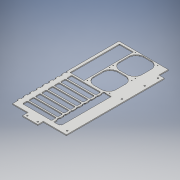
# Autodesk Inventor part: backpanel2
Saved by Autodesk Inventor 2018 (Build 220112000, 112)
## iProperties
Created: 2021-05-09
Part Number: backpanel2
Material: Generic
Document SubType Name: Modeling
Designer: gisen
Density: 1 g/cm^3
Appearance: Default
Author: gisen
Autodesk Inventor part; units mm, degrees
(part 1 of 2)
ref_plane "YZ Plane" through (0, 0, 0) normal (1, 0, 0) x (0, 1, 0)
ref_plane "XZ Plane" through (0, 0, 0) normal (0, 1, 0) x (-1, 0, 0)
ref_plane "XY Plane" through (0, 0, 0) normal (0, 0, 1) x (1, 0, 0)
sketch "Sketch2" plane through (0, 0, 0) normal (0, 0, 1) x (1, 0, 0)
  arc A0 (64.4142, -110.1237) -> (63.7071, -110.4166) centre (64.4142, -111.1237) ccw
  line L0 (63.7071, -110.4166) -> (59.2929, -114.8308)
  arc A1 (58.5858, -115.1237) -> (59.2929, -114.8308) centre (58.5858, -114.1237) ccw
  line L1 (58.5858, -115.1237) -> (43.2196, -115.1237)
  arc A2 (42.2196, -114.1237) -> (43.2196, -115.1237) centre (43.2196, -114.1237) ccw
  line L2 (42.2196, -114.1237) -> (42.2196, -104.6674)
  arc A3 (42.2196, -104.6674) -> (40.773, -102.7455) centre (40.2196, -104.6674) ccw
  arc A4 (39.7673, -102.1811) -> (40.773, -102.7455) centre (41.4696, -100.3262) ccw
  arc A5 (39.1196, -100.7076) -> (39.7673, -102.1811) centre (41.1196, -100.7076) ccw
  line L3 (39.1196, -100.7076) -> (39.1196, -95.7515)
  arc A6 (39.7673, -94.2779) -> (39.1196, -95.7515) centre (41.1196, -95.7515) ccw
  arc A7 (39.937, -94.1354) -> (39.7673, -94.2779) centre (41.4696, -96.1328) ccw
  arc A8 (39.937, -94.1354) -> (40.7196, -92.5486) centre (38.7196, -92.5486) ccw
  line L4 (40.7196, -92.5486) -> (40.7196, -83.4104)
  arc A9 (40.7196, -83.4104) -> (39.937, -81.8236) centre (38.7196, -83.4104) ccw
  arc A10 (39.7673, -81.6811) -> (39.937, -81.8236) centre (41.4696, -79.8262) ccw
  arc A11 (39.1196, -80.2076) -> (39.7673, -81.6811) centre (41.1196, -80.2076) ccw
  line L5 (39.1196, -80.2076) -> (39.1196, -75.2515)
  arc A12 (39.7673, -73.7779) -> (39.1196, -75.2515) centre (41.1196, -75.2515) ccw
  arc A13 (39.937, -73.6354) -> (39.7673, -73.7779) centre (41.4696, -75.6328) ccw
  arc A14 (39.937, -73.6354) -> (40.7196, -72.0486) centre (38.7196, -72.0486) ccw
  line L6 (40.7196, -72.0486) -> (40.7196, -62.9104)
  arc A15 (40.7196, -62.9104) -> (39.937, -61.3236) centre (38.7196, -62.9104) ccw
  arc A16 (39.7673, -61.1811) -> (39.937, -61.3236) centre (41.4696, -59.3262) ccw
  arc A17 (39.1196, -59.7076) -> (39.7673, -61.1811) centre (41.1196, -59.7076) ccw
  line L7 (39.1196, -59.7076) -> (39.1196, -54.7515)
  arc A18 (39.7673, -53.2779) -> (39.1196, -54.7515) centre (41.1196, -54.7515) ccw
  arc A19 (39.937, -53.1354) -> (39.7673, -53.2779) centre (41.4696, -55.1328) ccw
  arc A20 (39.937, -53.1354) -> (40.7196, -51.5486) centre (38.7196, -51.5486) ccw
  line L8 (40.7196, -51.5486) -> (40.7196, -42.4104)
  arc A21 (40.7196, -42.4104) -> (39.937, -40.8236) centre (38.7196, -42.4104) ccw
  arc A22 (39.7673, -40.6811) -> (39.937, -40.8236) centre (41.4696, -38.8262) ccw
  arc A23 (39.1196, -39.2076) -> (39.7673, -40.6811) centre (41.1196, -39.2076) ccw
  line L9 (39.1196, -39.2076) -> (39.1196, -34.2515)
  arc A24 (39.7673, -32.7779) -> (39.1196, -34.2515) centre (41.1196, -34.2515) ccw
  arc A25 (39.937, -32.6354) -> (39.7673, -32.7779) centre (41.4696, -34.6328) ccw
  arc A26 (39.937, -32.6354) -> (40.7196, -31.0486) centre (38.7196, -31.0486) ccw
  line L10 (40.7196, -31.0486) -> (40.7196, -21.9104)
  arc A27 (40.7196, -21.9104) -> (39.937, -20.3236) centre (38.7196, -21.9104) ccw
  arc A28 (39.7673, -20.1811) -> (39.937, -20.3236) centre (41.4696, -18.3262) ccw
  arc A29 (39.1196, -18.7076) -> (39.7673, -20.1811) centre (41.1196, -18.7076) ccw
  line L11 (39.1196, -18.7076) -> (39.1196, -13.7515)
  arc A30 (39.7673, -12.2779) -> (39.1196, -13.7515) centre (41.1196, -13.7515) ccw
  arc A31 (39.937, -12.1354) -> (39.7673, -12.2779) centre (41.4696, -14.1328) ccw
  arc A32 (39.937, -12.1354) -> (40.7196, -10.5486) centre (38.7196, -10.5486) ccw
  line L12 (40.7196, -10.5486) -> (40.7196, -1.4104)
  arc A33 (40.7196, -1.4104) -> (39.937, 0.1764) centre (38.7196, -1.4104) ccw
  arc A34 (39.7673, 0.3189) -> (39.937, 0.1764) centre (41.4696, 2.1738) ccw
  arc A35 (39.1196, 1.7924) -> (39.7673, 0.3189) centre (41.1196, 1.7924) ccw
  line L13 (39.1196, 1.7924) -> (39.1196, 6.7485)
  arc A36 (39.7673, 8.2221) -> (39.1196, 6.7485) centre (41.1196, 6.7485) ccw
  arc A37 (39.937, 8.3646) -> (39.7673, 8.2221) centre (41.4696, 6.3672) ccw
  arc A38 (39.937, 8.3646) -> (40.7196, 9.9514) centre (38.7196, 9.9514) ccw
  line L14 (40.7196, 9.9514) -> (40.7196, 19.0896)
  arc A39 (40.7196, 19.0896) -> (39.937, 20.6764) centre (38.7196, 19.0896) ccw
  arc A40 (39.7673, 20.8189) -> (39.937, 20.6764) centre (41.4696, 22.6738) ccw
  arc A41 (39.1196, 22.2924) -> (39.7673, 20.8189) centre (41.1196, 22.2924) ccw
  line L15 (39.1196, 22.2924) -> (39.1196, 27.2485)
  arc A42 (39.7673, 28.7221) -> (39.1196, 27.2485) centre (41.1196, 27.2485) ccw
  arc A43 (39.937, 28.8646) -> (39.7673, 28.7221) centre (41.4696, 26.8672) ccw
  arc A44 (39.937, 28.8646) -> (40.7196, 30.4514) centre (38.7196, 30.4514) ccw
  line L16 (40.7196, 30.4514) -> (40.7196, 39.5896)
  arc A45 (40.7196, 39.5896) -> (39.937, 41.1764) centre (38.7196, 39.5896) ccw
  arc A46 (39.7673, 41.3189) -> (39.937, 41.1764) centre (41.4696, 43.1738) ccw
  arc A47 (39.1196, 42.7924) -> (39.7673, 41.3189) centre (41.1196, 42.7924) ccw
  line L17 (39.1196, 42.7924) -> (39.1196, 47.7485)
  arc A48 (39.7673, 49.2221) -> (39.1196, 47.7485) centre (41.1196, 47.7485) ccw
  arc A49 (43.3362, 49.0566) -> (39.7673, 49.2221) centre (41.4696, 47.3672) ccw
  arc A50 (43.3362, 49.0566) -> (44.819, 48.3987) centre (44.819, 50.3987) ccw
  line L18 (44.819, 48.3987) -> (75, 48.3987)
  line L19 (75, 48.3987) -> (75, 184.5)
  line L20 (75, 184.5) -> (57.5, 184.5)
  line L21 (57.5, 184.5) -> (57.5, 215)
  line L22 (57.5, 215) -> (55, 215)
  line L23 (55, 215) -> (55, 220)
  line L24 (55, 220) -> (24.5, 220)
  line L25 (24.5, 220) -> (24.5, 232.5)
  line L26 (24.5, 232.5) -> (-24.5, 232.5)
  line L27 (-24.5, 232.5) -> (-24.5, 220)
  line L28 (-24.5, 220) -> (-55, 220)
  line L29 (-55, 220) -> (-55, 215)
  line L30 (-55, 215) -> (-78, 215)
  line L31 (-78, 215) -> (-78, 46.0635)
  line L32 (-78, 46.0635) -> (-75, 46.0635)
  line L33 (-75, 46.0635) -> (-75, 40.8932)
  line L34 (-75, 40.8932) -> (-78, 40.8932)
  line L35 (-78, 40.8932) -> (-78, 30.6062)
  line L36 (-78, 30.6062) -> (-75, 30.6062)
  line L37 (-75, 30.6062) -> (-75, 20.5478)
  line L38 (-75, 20.5478) -> (-78, 20.5478)
  line L39 (-78, 20.5478) -> (-78, 10.2608)
  line L40 (-78, 10.2608) -> (-75, 10.2608)
  line L41 (-75, 10.2608) -> (-75, -0.1068)
  line L42 (-75, -0.1068) -> (-78, -0.1068)
  line L43 (-78, -0.1068) -> (-78, -10.3938)
  line L44 (-78, -10.3938) -> (-75, -10.3938)
  line L45 (-75, -10.3938) -> (-75, -20.4522)
  line L46 (-75, -20.4522) -> (-78, -20.4522)
  line L47 (-78, -20.4522) -> (-78, -30.7392)
  line L48 (-78, -30.7392) -> (-75, -30.7392)
  line L49 (-75, -30.7392) -> (-75, -41.1068)
  line L50 (-75, -41.1068) -> (-78, -41.1068)
  line L51 (-78, -41.1068) -> (-78, -51.3938)
  line L52 (-78, -51.3938) -> (-75, -51.3938)
  line L53 (-75, -51.3938) -> (-75, -61.4522)
  line L54 (-75, -61.4522) -> (-78, -61.4522)
  line L55 (-78, -61.4522) -> (-78, -71.7392)
  line L56 (-78, -71.7392) -> (-75, -71.7392)
  line L57 (-75, -71.7392) -> (-75, -82.1068)
  line L58 (-75, -82.1068) -> (-78, -82.1068)
  line L59 (-78, -82.1068) -> (-78, -92.3938)
  line L60 (-78, -92.3938) -> (-75, -92.3938)
  line L61 (-75, -92.3938) -> (-75, -102.4522)
  line L62 (-75, -102.4522) -> (-78, -102.4522)
  line L63 (-78, -102.4522) -> (-78, -112.7392)
  line L64 (-55.8933, -130) -> (-55.8933, -135)
  line L65 (-55.8933, -135) -> (-25.3933, -135)
  line L66 (-25.3933, -135) -> (-25.3933, -147.5)
  line L67 (-25.3933, -147.5) -> (23.6067, -147.5)
  line L68 (23.6067, -147.5) -> (23.6067, -135)
  line L69 (23.6067, -135) -> (54.1067, -135)
  line L70 (54.1067, -135) -> (54.1067, -130)
  line L71 (75, -115.1237) -> (75, -111.1237)
  arc A51 (75, -111.1237) -> (74, -110.1237) centre (74, -111.1237) ccw
  line L72 (74, -110.1237) -> (64.4142, -110.1237)
  arc A52 (39.7304, 54.8876) -> (46.6028, 60.5179) centre (16.3806, 90.3987) ccw
  arc A53 (28.7422, 51.5987) -> (39.7304, 54.8876) centre (28.7422, 71.5987) ccw
  line L73 (28.7422, 51.5987) -> (4.019, 51.5987)
  arc A54 (-6.9692, 54.8876) -> (4.019, 51.5987) centre (4.019, 71.5987) ccw
  arc A55 (-13.8416, 60.5179) -> (-6.9692, 54.8876) centre (16.3806, 90.3987) ccw
  arc A56 (-19.6194, 74.5794) -> (-13.8416, 60.5179) centre (0.3806, 74.5794) ccw
  line L74 (-19.6194, 74.5794) -> (-19.6194, 106.218)
  arc A57 (-13.8416, 120.2796) -> (-19.6194, 106.218) centre (0.3806, 106.218) ccw
  arc A58 (-6.9692, 125.9099) -> (-13.8416, 120.2796) centre (16.3806, 90.3987) ccw
  arc A59 (4.019, 129.1987) -> (-6.9692, 125.9099) centre (4.019, 109.1987) ccw
  line L75 (4.019, 129.1987) -> (28.7422, 129.1987)
  arc A60 (39.7304, 125.9099) -> (28.7422, 129.1987) centre (28.7422, 109.1987) ccw
  arc A61 (46.6028, 120.2796) -> (39.7304, 125.9099) centre (16.3806, 90.3987) ccw
  arc A62 (52.3806, 106.218) -> (46.6028, 120.2796) centre (32.3806, 106.218) ccw
  line L76 (52.3806, 74.5794) -> (52.3806, 106.218)
  arc A63 (46.6028, 60.5179) -> (52.3806, 74.5794) centre (32.3806, 74.5794) ccw
  circle A64 centre (52.1306, 137.6487) radius 1.2
  circle A65 centre (-19.3694, 209.1487) radius 1.2
  circle A66 centre (-19.3694, 54.6487) radius 1.2
  circle A67 centre (-19.3694, 126.1487) radius 1.2
  circle A68 centre (52.1306, 126.1487) radius 1.2
  circle A69 centre (52.1306, 54.6487) radius 1.2
  circle A70 centre (52.1306, 209.1487) radius 1.2
  circle A71 centre (-19.3694, 137.6487) radius 1.2
  arc A72 (39.7304, 137.8876) -> (46.6028, 143.5179) centre (16.3806, 173.3987) ccw
  arc A73 (28.7422, 134.5987) -> (39.7304, 137.8876) centre (28.7422, 154.5987) ccw
  line L77 (28.7422, 134.5987) -> (4.019, 134.5987)
  arc A74 (-6.9692, 137.8876) -> (4.019, 134.5987) centre (4.019, 154.5987) ccw
  arc A75 (-13.8416, 143.5179) -> (-6.9692, 137.8876) centre (16.3806, 173.3987) ccw
  arc A76 (-19.6194, 157.5794) -> (-13.8416, 143.5179) centre (0.3806, 157.5794) ccw
  line L78 (-19.6194, 157.5794) -> (-19.6194, 189.218)
  arc A77 (-13.8416, 203.2796) -> (-19.6194, 189.218) centre (0.3806, 189.218) ccw
  arc A78 (-6.9692, 208.9099) -> (-13.8416, 203.2796) centre (16.3806, 173.3987) ccw
  arc A79 (4.019, 212.1987) -> (-6.9692, 208.9099) centre (4.019, 192.1987) ccw
  line L79 (4.019, 212.1987) -> (28.7422, 212.1987)
  arc A80 (39.7304, 208.9099) -> (28.7422, 212.1987) centre (28.7422, 192.1987) ccw
  arc A81 (46.6028, 203.2796) -> (39.7304, 208.9099) centre (16.3806, 173.3987) ccw
  arc A82 (52.3806, 189.218) -> (46.6028, 203.2796) centre (32.3806, 189.218) ccw
  line L80 (52.3806, 157.5794) -> (52.3806, 189.218)
  arc A83 (46.6028, 143.5179) -> (52.3806, 157.5794) centre (32.3806, 157.5794) ccw
  line L81 (-24.6194, 207.0635) -> (-24.6194, 50.0635)
  arc A84 (-25.6194, 49.0635) -> (-24.6194, 50.0635) centre (-25.6194, 50.0635) ccw
  line L82 (-25.6194, 49.0635) -> (-68.3194, 49.0635)
  arc A85 (-69.3194, 50.0635) -> (-68.3194, 49.0635) centre (-68.3194, 50.0635) ccw
  line L83 (-69.3194, 50.0635) -> (-69.3194, 207.0635)
  arc A86 (-68.3194, 208.0635) -> (-69.3194, 207.0635) centre (-68.3194, 207.0635) ccw
  line L84 (-68.3194, 208.0635) -> (-25.6194, 208.0635)
  arc A87 (-24.6194, 207.0635) -> (-25.6194, 208.0635) centre (-25.6194, 207.0635) ccw
  line L85 (34.7396, -81.3827) -> (34.7396, -91.2627)
  arc A88 (31.7396, -94.2627) -> (34.7396, -91.2627) centre (31.7396, -91.2627) ccw
  line L86 (31.7396, -94.2627) -> (-55.9404, -94.2627)
  arc A89 (-58.9404, -91.2627) -> (-55.9404, -94.2627) centre (-55.9404, -91.2627) ccw
  line L87 (-58.9404, -91.2627) -> (-58.9404, -81.3827)
  arc A90 (-55.9404, -78.3827) -> (-58.9404, -81.3827) centre (-55.9404, -81.3827) ccw
  line L88 (-55.9404, -78.3827) -> (31.7396, -78.3827)
  arc A91 (34.7396, -81.3827) -> (31.7396, -78.3827) centre (31.7396, -81.3827) ccw
  line L89 (34.7396, -40.6919) -> (34.7396, -50.5719)
  arc A92 (31.7396, -53.5719) -> (34.7396, -50.5719) centre (31.7396, -50.5719) ccw
  line L90 (31.7396, -53.5719) -> (-55.9404, -53.5719)
  arc A93 (-58.9404, -50.5719) -> (-55.9404, -53.5719) centre (-55.9404, -50.5719) ccw
  line L91 (-58.9404, -50.5719) -> (-58.9404, -40.6919)
  arc A94 (-55.9404, -37.6919) -> (-58.9404, -40.6919) centre (-55.9404, -40.6919) ccw
  line L92 (-55.9404, -37.6919) -> (31.7396, -37.6919)
  arc A95 (34.7396, -40.6919) -> (31.7396, -37.6919) centre (31.7396, -40.6919) ccw
  line L93 (34.7396, -0.0011) -> (34.7396, -9.8811)
  arc A96 (31.7396, -12.8811) -> (34.7396, -9.8811) centre (31.7396, -9.8811) ccw
  line L94 (31.7396, -12.8811) -> (-55.9404, -12.8811)
  arc A97 (-58.9404, -9.8811) -> (-55.9404, -12.8811) centre (-55.9404, -9.8811) ccw
  line L95 (-58.9404, -9.8811) -> (-58.9404, -0.0011)
  arc A98 (-55.9404, 2.9989) -> (-58.9404, -0.0011) centre (-55.9404, -0.0011) ccw
  line L96 (-55.9404, 2.9989) -> (31.7396, 2.9989)
  arc A99 (34.7396, -0.0011) -> (31.7396, 2.9989) centre (31.7396, -0.0011) ccw
  line L97 (34.7396, 40.6897) -> (34.7396, 30.8097)
  arc A100 (31.7396, 27.8097) -> (34.7396, 30.8097) centre (31.7396, 30.8097) ccw
  line L98 (31.7396, 27.8097) -> (-55.9404, 27.8097)
  arc A101 (-58.9404, 30.8097) -> (-55.9404, 27.8097) centre (-55.9404, 30.8097) ccw
  line L99 (-58.9404, 30.8097) -> (-58.9404, 40.6897)
  arc A102 (-55.9404, 43.6897) -> (-58.9404, 40.6897) centre (-55.9404, 40.6897) ccw
  line L100 (-55.9404, 43.6897) -> (31.7396, 43.6897)
  arc A103 (34.7396, 40.6897) -> (31.7396, 43.6897) centre (31.7396, 40.6897) ccw
  line L101 (34.7396, 20.3443) -> (34.7396, 10.4643)
  arc A104 (31.7396, 7.4643) -> (34.7396, 10.4643) centre (31.7396, 10.4643) ccw
  line L102 (31.7396, 7.4643) -> (-55.9404, 7.4643)
  arc A105 (-58.9404, 10.4643) -> (-55.9404, 7.4643) centre (-55.9404, 10.4643) ccw
  line L103 (-58.9404, 10.4643) -> (-58.9404, 20.3443)
  arc A106 (-55.9404, 23.3443) -> (-58.9404, 20.3443) centre (-55.9404, 20.3443) ccw
  line L104 (-55.9404, 23.3443) -> (31.7396, 23.3443)
  arc A107 (34.7396, 20.3443) -> (31.7396, 23.3443) centre (31.7396, 20.3443) ccw
  line L105 (34.7396, -20.3465) -> (34.7396, -30.2265)
  arc A108 (31.7396, -33.2265) -> (34.7396, -30.2265) centre (31.7396, -30.2265) ccw
  line L106 (31.7396, -33.2265) -> (-55.9404, -33.2265)
  arc A109 (-58.9404, -30.2265) -> (-55.9404, -33.2265) centre (-55.9404, -30.2265) ccw
  line L107 (-58.9404, -30.2265) -> (-58.9404, -20.3465)
  arc A110 (-55.9404, -17.3465) -> (-58.9404, -20.3465) centre (-55.9404, -20.3465) ccw
  line L108 (-55.9404, -17.3465) -> (31.7396, -17.3465)
  arc A111 (34.7396, -20.3465) -> (31.7396, -17.3465) centre (31.7396, -20.3465) ccw
  line L109 (34.7396, -61.0373) -> (34.7396, -70.9173)
  arc A112 (31.7396, -73.9173) -> (34.7396, -70.9173) centre (31.7396, -70.9173) ccw
  line L110 (31.7396, -73.9173) -> (-55.9404, -73.9173)
  arc A113 (-58.9404, -70.9173) -> (-55.9404, -73.9173) centre (-55.9404, -70.9173) ccw
  line L111 (-58.9404, -70.9173) -> (-58.9404, -61.0373)
  arc A114 (-55.9404, -58.0373) -> (-58.9404, -61.0373) centre (-55.9404, -61.0373) ccw
  line L112 (-55.9404, -58.0373) -> (31.7396, -58.0373)
  arc A115 (34.7396, -61.0373) -> (31.7396, -58.0373) centre (31.7396, -61.0373) ccw
  line L113 (34.7396, -101.7281) -> (34.7396, -111.6081)
  arc A116 (31.7396, -114.6081) -> (34.7396, -111.6081) centre (31.7396, -111.6081) ccw
  line L114 (31.7396, -114.6081) -> (-55.9404, -114.6081)
  arc A117 (-58.9404, -111.6081) -> (-55.9404, -114.6081) centre (-55.9404, -111.6081) ccw
  line L115 (-58.9404, -111.6081) -> (-58.9404, -101.7281)
  arc A118 (-55.9404, -98.7281) -> (-58.9404, -101.7281) centre (-55.9404, -101.7281) ccw
  line L116 (-55.9404, -98.7281) -> (31.7396, -98.7281)
  arc A119 (34.7396, -101.7281) -> (31.7396, -98.7281) centre (31.7396, -101.7281) ccw
  circle A120 centre (16.1067, -140) radius 2.25
  circle A121 centre (-17, 225) radius 2.25
  circle A122 centre (65, 131.8987) radius 2.25
  circle A123 centre (65, 58.3987) radius 2.25
  circle A124 centre (17, 225) radius 2.25
  circle A125 centre (65, 174.5) radius 2.25
  circle A126 centre (-17.8933, -140) radius 2.25
  circle A127 centre (65, -117.6237) radius 2.25
  line L117 (-78, -112.7392) -> (-78, -115.1237)
  line L118 (-78, -115.1237) -> (-78, -130)
  line L119 (-78, -130) -> (-55.8933, -130)
  line L120 (54.1067, -130) -> (75, -130)
  line L121 (75, -130) -> (75, -115.1237)
  point P0 (0, 0)
  point P1 (0, 0)
  dimension "d17" = 232.5
  dimension "d19" = 7.5
  dimension "d20" = 7.5
  dimension "d22" = 49
  dimension "d23" = 12.5
  dimension "d24" = 30.5
  dimension "d26" = 7.5
  dimension "d27" = 7.5
  dimension "d28" = 12.5
  dimension "d29" = 30.5
  dimension "d33" = 380
  dimension "d35" = 12.5
  dimension "d36" = 12.5
  constraints: 244 end point, 224 point on circle, 128 centre point, 3 point on line, 2 perpendicular, 2 vertical
  measures "d17" distance from line of point (0, 0) L26
  measures "d19" distance from line of A126.centre L67
  measures "d20" distance from line of L67 A120.centre
  measures "d22" distance of L66.end L67.end
  measures "d23" distance of L65.end L66.end
  measures "d24" distance of L65.start L65.end
  measures "d26" distance from line of L66 A126.centre
  measures "d27" distance from line of A120.centre L68
  measures "d28" distance of L67.end L69.start
  measures "d29" distance of L69.start L69.end
  measures "d33" distance between parallel lines of L67 L26
  measures "d35" distance of L24.end L25.end
  measures "d36" distance of L26.end L27.end
extrude "Extrusion2" add sketch "Sketch2" along normal blind 3
sketch "Sketch3" plane through (0, 0, 3) normal (0, 0, 1) x (1, 0, 0)
  line L0 (-69.3194, 50.0635) -> (-69.3194, 207.0635) projected
  arc A0 (-68.3194, 208.0635) -> (-69.3194, 207.0635) centre (-68.3194, 207.0635) ccw projected
  line L1 (-68.3194, 208.0635) -> (-25.6194, 208.0635) projected
  arc A1 (-24.6194, 207.0635) -> (-25.6194, 208.0635) centre (-25.6194, 207.0635) ccw projected
  line L2 (-24.6194, 207.0635) -> (-24.6194, 50.0635) projected
  arc A2 (-25.6194, 49.0635) -> (-24.6194, 50.0635) centre (-25.6194, 50.0635) ccw projected
  line L3 (-25.6194, 49.0635) -> (-68.3194, 49.0635) projected
  arc A3 (-69.3194, 50.0635) -> (-68.3194, 49.0635) centre (-68.3194, 50.0635) ccw projected
  arc A4 (-6.9692, 137.8876) -> (4.019, 134.5987) centre (4.019, 154.5987) ccw projected
  arc A5 (-13.8416, 143.5179) -> (-6.9692, 137.8876) centre (16.3806, 173.3987) ccw projected
  arc A6 (-19.6194, 157.5794) -> (-13.8416, 143.5179) centre (0.3806, 157.5794) ccw projected
  line L4 (-19.6194, 157.5794) -> (-19.6194, 189.218) projected
  arc A7 (-13.8416, 203.2796) -> (-19.6194, 189.218) centre (0.3806, 189.218) ccw projected
  arc A8 (-6.9692, 208.9099) -> (-13.8416, 203.2796) centre (16.3806, 173.3987) ccw projected
  arc A9 (4.019, 212.1987) -> (-6.9692, 208.9099) centre (4.019, 192.1987) ccw projected
  line L5 (4.019, 212.1987) -> (28.7422, 212.1987) projected
  arc A10 (39.7304, 208.9099) -> (28.7422, 212.1987) centre (28.7422, 192.1987) ccw projected
  arc A11 (46.6028, 203.2796) -> (39.7304, 208.9099) centre (16.3806, 173.3987) ccw projected
  arc A12 (52.3806, 189.218) -> (46.6028, 203.2796) centre (32.3806, 189.218) ccw projected
  line L6 (52.3806, 189.218) -> (52.3806, 157.5794) projected
  arc A13 (46.6028, 143.5179) -> (52.3806, 157.5794) centre (32.3806, 157.5794) ccw projected
  arc A14 (39.7304, 137.8876) -> (46.6028, 143.5179) centre (16.3806, 173.3987) ccw projected
  arc A15 (28.7422, 134.5987) -> (39.7304, 137.8876) centre (28.7422, 154.5987) ccw projected
  line L7 (28.7422, 134.5987) -> (4.019, 134.5987) projected
  arc A16 (-6.9692, 54.8876) -> (4.019, 51.5987) centre (4.019, 71.5987) ccw projected
  arc A17 (-13.8416, 60.5179) -> (-6.9692, 54.8876) centre (16.3806, 90.3987) ccw projected
  arc A18 (-19.6194, 74.5794) -> (-13.8416, 60.5179) centre (0.3806, 74.5794) ccw projected
  line L8 (-19.6194, 74.5794) -> (-19.6194, 106.218) projected
  arc A19 (-13.8416, 120.2796) -> (-19.6194, 106.218) centre (0.3806, 106.218) ccw projected
  arc A20 (-6.9692, 125.9099) -> (-13.8416, 120.2796) centre (16.3806, 90.3987) ccw projected
  arc A21 (4.019, 129.1987) -> (-6.9692, 125.9099) centre (4.019, 109.1987) ccw projected
  line L9 (4.019, 129.1987) -> (28.7422, 129.1987) projected
  arc A22 (39.7304, 125.9099) -> (28.7422, 129.1987) centre (28.7422, 109.1987) ccw projected
  arc A23 (46.6028, 120.2796) -> (39.7304, 125.9099) centre (16.3806, 90.3987) ccw projected
  arc A24 (52.3806, 106.218) -> (46.6028, 120.2796) centre (32.3806, 106.218) ccw projected
  line L10 (52.3806, 106.218) -> (52.3806, 74.5794) projected
  arc A25 (46.6028, 60.5179) -> (52.3806, 74.5794) centre (32.3806, 74.5794) ccw projected
  arc A26 (39.7304, 54.8876) -> (46.6028, 60.5179) centre (16.3806, 90.3987) ccw projected
  arc A27 (28.7422, 51.5987) -> (39.7304, 54.8876) centre (28.7422, 71.5987) ccw projected
  line L11 (28.7422, 51.5987) -> (4.019, 51.5987) projected
  arc A28 (31.7396, -114.6081) -> (34.7396, -111.6081) centre (31.7396, -111.6081) ccw projected
  line L12 (31.7396, -114.6081) -> (-55.9404, -114.6081) projected
  arc A29 (-58.9404, -111.6081) -> (-55.9404, -114.6081) centre (-55.9404, -111.6081) ccw projected
  line L13 (-58.9404, -111.6081) -> (-58.9404, -101.7281) projected
  arc A30 (-55.9404, -98.7281) -> (-58.9404, -101.7281) centre (-55.9404, -101.7281) ccw projected
  line L14 (-55.9404, -98.7281) -> (31.7396, -98.7281) projected
  arc A31 (34.7396, -101.7281) -> (31.7396, -98.7281) centre (31.7396, -101.7281) ccw projected
  line L15 (34.7396, -101.7281) -> (34.7396, -111.6081) projected
  arc A32 (34.7396, -81.3827) -> (31.7396, -78.3827) centre (31.7396, -81.3827) ccw projected
  line L16 (34.7396, -81.3827) -> (34.7396, -91.2627) projected
  arc A33 (31.7396, -94.2627) -> (34.7396, -91.2627) centre (31.7396, -91.2627) ccw projected
  line L17 (31.7396, -94.2627) -> (-55.9404, -94.2627) projected
  arc A34 (-58.9404, -91.2627) -> (-55.9404, -94.2627) centre (-55.9404, -91.2627) ccw projected
  line L18 (-58.9404, -91.2627) -> (-58.9404, -81.3827) projected
  arc A35 (-55.9404, -78.3827) -> (-58.9404, -81.3827) centre (-55.9404, -81.3827) ccw projected
  line L19 (-55.9404, -78.3827) -> (31.7396, -78.3827) projected
  line L20 (31.7396, -33.2265) -> (-55.9404, -33.2265) projected
  arc A36 (-58.9404, -30.2265) -> (-55.9404, -33.2265) centre (-55.9404, -30.2265) ccw projected
  line L21 (-58.9404, -30.2265) -> (-58.9404, -20.3465) projected
  arc A37 (-55.9404, -17.3465) -> (-58.9404, -20.3465) centre (-55.9404, -20.3465) ccw projected
  line L22 (-55.9404, -17.3465) -> (31.7396, -17.3465) projected
  arc A38 (34.7396, -20.3465) -> (31.7396, -17.3465) centre (31.7396, -20.3465) ccw projected
  line L23 (34.7396, -20.3465) -> (34.7396, -30.2265) projected
  arc A39 (31.7396, -33.2265) -> (34.7396, -30.2265) centre (31.7396, -30.2265) ccw projected
  line L24 (-55.9404, -58.0373) -> (31.7396, -58.0373) projected
  arc A40 (34.7396, -61.0373) -> (31.7396, -58.0373) centre (31.7396, -61.0373) ccw projected
  line L25 (34.7396, -61.0373) -> (34.7396, -70.9173) projected
  arc A41 (31.7396, -73.9173) -> (34.7396, -70.9173) centre (31.7396, -70.9173) ccw projected
  line L26 (31.7396, -73.9173) -> (-55.9404, -73.9173) projected
  arc A42 (-58.9404, -70.9173) -> (-55.9404, -73.9173) centre (-55.9404, -70.9173) ccw projected
  line L27 (-58.9404, -70.9173) -> (-58.9404, -61.0373) projected
  arc A43 (-55.9404, -58.0373) -> (-58.9404, -61.0373) centre (-55.9404, -61.0373) ccw projected
  arc A44 (-55.9404, -37.6919) -> (-58.9404, -40.6919) centre (-55.9404, -40.6919) ccw projected
  line L28 (-55.9404, -37.6919) -> (31.7396, -37.6919) projected
  arc A45 (34.7396, -40.6919) -> (31.7396, -37.6919) centre (31.7396, -40.6919) ccw projected
  line L29 (34.7396, -40.6919) -> (34.7396, -50.5719) projected
  arc A46 (31.7396, -53.5719) -> (34.7396, -50.5719) centre (31.7396, -50.5719) ccw projected
  line L30 (31.7396, -53.5719) -> (-55.9404, -53.5719) projected
  arc A47 (-58.9404, -50.5719) -> (-55.9404, -53.5719) centre (-55.9404, -50.5719) ccw projected
  line L31 (-58.9404, -50.5719) -> (-58.9404, -40.6919) projected
  arc A48 (-55.9404, 2.9989) -> (-58.9404, -0.0011) centre (-55.9404, -0.0011) ccw projected
  line L32 (-55.9404, 2.9989) -> (31.7396, 2.9989) projected
  arc A49 (34.7396, -0.0011) -> (31.7396, 2.9989) centre (31.7396, -0.0011) ccw projected
  line L33 (34.7396, -0.0011) -> (34.7396, -9.8811) projected
  arc A50 (31.7396, -12.8811) -> (34.7396, -9.8811) centre (31.7396, -9.8811) ccw projected
  line L34 (31.7396, -12.8811) -> (-55.9404, -12.8811) projected
  arc A51 (-58.9404, -9.8811) -> (-55.9404, -12.8811) centre (-55.9404, -9.8811) ccw projected
  line L35 (-58.9404, -9.8811) -> (-58.9404, -0.0011) projected
  line L36 (-58.9404, 30.8097) -> (-58.9404, 40.6897) projected
  arc A52 (-55.9404, 43.6897) -> (-58.9404, 40.6897) centre (-55.9404, 40.6897) ccw projected
  line L37 (-55.9404, 43.6897) -> (31.7396, 43.6897) projected
  arc A53 (34.7396, 40.6897) -> (31.7396, 43.6897) centre (31.7396, 40.6897) ccw projected
  line L38 (34.7396, 40.6897) -> (34.7396, 30.8097) projected
  arc A54 (31.7396, 27.8097) -> (34.7396, 30.8097) centre (31.7396, 30.8097) ccw projected
  line L39 (31.7396, 27.8097) -> (-55.9404, 27.8097) projected
  arc A55 (-58.9404, 30.8097) -> (-55.9404, 27.8097) centre (-55.9404, 30.8097) ccw projected
  line L40 (-58.9404, 10.4643) -> (-58.9404, 20.3443) projected
  arc A56 (-55.9404, 23.3443) -> (-58.9404, 20.3443) centre (-55.9404, 20.3443) ccw projected
  line L41 (-55.9404, 23.3443) -> (31.7396, 23.3443) projected
  arc A57 (34.7396, 20.3443) -> (31.7396, 23.3443) centre (31.7396, 20.3443) ccw projected
  line L42 (34.7396, 20.3443) -> (34.7396, 10.4643) projected
  arc A58 (31.7396, 7.4643) -> (34.7396, 10.4643) centre (31.7396, 10.4643) ccw projected
  line L43 (31.7396, 7.4643) -> (-55.9404, 7.4643) projected
  arc A59 (-58.9404, 10.4643) -> (-55.9404, 7.4643) centre (-55.9404, 10.4643) ccw projected
  circle A60 centre (16.1067, -140) radius 2.25 projected
  circle A61 centre (-17.8933, -140) radius 2.25 projected
  circle A62 centre (65, -117.6237) radius 2.25 projected
  circle A63 centre (-17, 225) radius 2.25 projected
  circle A64 centre (17, 225) radius 2.25 projected
  circle A65 centre (65, 174.5) radius 2.25 projected
  circle A66 centre (65, 131.8987) radius 2.25 projected
  circle A67 centre (65, 58.3987) radius 2.25 projected
  circle A68 centre (-19.3694, 54.6487) radius 1.2 projected
  circle A69 centre (-19.3694, 209.1487) radius 1.2 projected
  circle A70 centre (-19.3694, 137.6487) radius 1.2 projected
  circle A71 centre (52.1306, 54.6487) radius 1.2 projected
  circle A72 centre (52.1306, 209.1487) radius 1.2 projected
  circle A73 centre (52.1306, 137.6487) radius 1.2 projected
  circle A74 centre (52.1306, 126.1487) radius 1.2 projected
  circle A75 centre (-19.3694, 126.1487) radius 1.2 projected
  line L44 (-75, 46.0635) -> (-75, 40.8932) projected
  line L45 (-75, 40.8932) -> (-78, 40.8932) projected
  line L46 (-78, 40.8932) -> (-78, 30.6062) projected
  line L47 (-78, 30.6062) -> (-75, 30.6062) projected
  line L48 (-75, 30.6062) -> (-75, 20.5478) projected
  line L49 (-75, 20.5478) -> (-78, 20.5478) projected
  line L50 (-78, 20.5478) -> (-78, 10.2608) projected
  line L51 (-78, 10.2608) -> (-75, 10.2608) projected
  line L52 (-75, 10.2608) -> (-75, -0.1068) projected
  line L53 (-75, -0.1068) -> (-78, -0.1068) projected
  line L54 (-78, -0.1068) -> (-78, -10.3938) projected
  line L55 (-78, -10.3938) -> (-75, -10.3938) projected
  line L56 (-75, -10.3938) -> (-75, -20.4522) projected
  line L57 (-75, -20.4522) -> (-78, -20.4522) projected
  line L58 (-78, -20.4522) -> (-78, -30.7392) projected
  line L59 (-78, -30.7392) -> (-75, -30.7392) projected
  line L60 (-75, -30.7392) -> (-75, -41.1068) projected
  line L61 (-75, -41.1068) -> (-78, -41.1068) projected
  line L62 (-78, -41.1068) -> (-78, -51.3938) projected
  line L63 (-78, -51.3938) -> (-75, -51.3938) projected
  line L64 (-75, -51.3938) -> (-75, -61.4522) projected
  line L65 (-75, -61.4522) -> (-78, -61.4522) projected
  line L66 (-78, -61.4522) -> (-78, -71.7392) projected
  line L67 (-78, -71.7392) -> (-75, -71.7392) projected
  line L68 (-75, -71.7392) -> (-75, -82.1068) projected
  line L69 (-75, -82.1068) -> (-78, -82.1068) projected
  line L70 (-78, -82.1068) -> (-78, -92.3938) projected
  line L71 (-78, -92.3938) -> (-75, -92.3938) projected
  line L72 (-75, -92.3938) -> (-75, -102.4522) projected
  line L73 (-75, -102.4522) -> (-78, -102.4522) projected
  line L74 (-78, -102.4522) -> (-78, -130) projected
  line L75 (-78, -130) -> (-55.8933, -130) projected
  line L76 (-55.8933, -130) -> (-55.8933, -135) projected
  line L77 (-55.8933, -135) -> (-25.3933, -135) projected
  line L78 (-25.3933, -135) -> (-25.3933, -147.5) projected
  line L79 (-25.3933, -147.5) -> (23.6067, -147.5) projected
  line L80 (23.6067, -147.5) -> (23.6067, -135) projected
  line L81 (23.6067, -135) -> (54.1067, -135) projected
  line L82 (54.1067, -135) -> (54.1067, -130) projected
  line L83 (54.1067, -130) -> (75, -130) projected
  line L84 (75, -130) -> (75, -111.1237) projected
  arc A76 (75, -111.1237) -> (74, -110.1237) centre (74, -111.1237) ccw projected
  line L85 (74, -110.1237) -> (64.4142, -110.1237) projected
  arc A77 (64.4142, -110.1237) -> (63.7071, -110.4166) centre (64.4142, -111.1237) ccw projected
  line L86 (63.7071, -110.4166) -> (59.2929, -114.8308) projected
  arc A78 (58.5858, -115.1237) -> (59.2929, -114.8308) centre (58.5858, -114.1237) ccw projected
  line L87 (58.5858, -115.1237) -> (43.2196, -115.1237) projected
  arc A79 (42.2196, -114.1237) -> (43.2196, -115.1237) centre (43.2196, -114.1237) ccw projected
  line L88 (42.2196, -114.1237) -> (42.2196, -104.6674) projected
  arc A80 (42.2196, -104.6674) -> (40.773, -102.7455) centre (40.2196, -104.6674) ccw projected
  arc A81 (39.7673, -102.1811) -> (40.773, -102.7455) centre (41.4696, -100.3262) ccw projected
  arc A82 (39.1196, -100.7076) -> (39.7673, -102.1811) centre (41.1196, -100.7076) ccw projected
  line L89 (39.1196, -100.7076) -> (39.1196, -95.7515) projected
  arc A83 (39.7673, -94.2779) -> (39.1196, -95.7515) centre (41.1196, -95.7515) ccw projected
  arc A84 (39.937, -94.1354) -> (39.7673, -94.2779) centre (41.4696, -96.1328) ccw projected
  arc A85 (39.937, -94.1354) -> (40.7196, -92.5486) centre (38.7196, -92.5486) ccw projected
  line L90 (40.7196, -92.5486) -> (40.7196, -83.4104) projected
  arc A86 (40.7196, -83.4104) -> (39.937, -81.8236) centre (38.7196, -83.4104) ccw projected
  arc A87 (39.7673, -81.6811) -> (39.937, -81.8236) centre (41.4696, -79.8262) ccw projected
  arc A88 (39.1196, -80.2076) -> (39.7673, -81.6811) centre (41.1196, -80.2076) ccw projected
  line L91 (39.1196, -80.2076) -> (39.1196, -75.2515) projected
  arc A89 (39.7673, -73.7779) -> (39.1196, -75.2515) centre (41.1196, -75.2515) ccw projected
  arc A90 (39.937, -73.6354) -> (39.7673, -73.7779) centre (41.4696, -75.6328) ccw projected
  arc A91 (39.937, -73.6354) -> (40.7196, -72.0486) centre (38.7196, -72.0486) ccw projected
  line L92 (40.7196, -72.0486) -> (40.7196, -62.9104) projected
  arc A92 (40.7196, -62.9104) -> (39.937, -61.3236) centre (38.7196, -62.9104) ccw projected
  arc A93 (39.7673, -61.1811) -> (39.937, -61.3236) centre (41.4696, -59.3262) ccw projected
  arc A94 (39.1196, -59.7076) -> (39.7673, -61.1811) centre (41.1196, -59.7076) ccw projected
  line L93 (39.1196, -59.7076) -> (39.1196, -54.7515) projected
  arc A95 (39.7673, -53.2779) -> (39.1196, -54.7515) centre (41.1196, -54.7515) ccw projected
  arc A96 (39.937, -53.1354) -> (39.7673, -53.2779) centre (41.4696, -55.1328) ccw projected
  arc A97 (39.937, -53.1354) -> (40.7196, -51.5486) centre (38.7196, -51.5486) ccw projected
  line L94 (40.7196, -51.5486) -> (40.7196, -42.4104) projected
  arc A98 (40.7196, -42.4104) -> (39.937, -40.8236) centre (38.7196, -42.4104) ccw projected
  arc A99 (39.7673, -40.6811) -> (39.937, -40.8236) centre (41.4696, -38.8262) ccw projected
  arc A100 (39.1196, -39.2076) -> (39.7673, -40.6811) centre (41.1196, -39.2076) ccw projected
  line L95 (39.1196, -39.2076) -> (39.1196, -34.2515) projected
  arc A101 (39.7673, -32.7779) -> (39.1196, -34.2515) centre (41.1196, -34.2515) ccw projected
  arc A102 (39.937, -32.6354) -> (39.7673, -32.7779) centre (41.4696, -34.6328) ccw projected
  arc A103 (39.937, -32.6354) -> (40.7196, -31.0486) centre (38.7196, -31.0486) ccw projected
  line L96 (40.7196, -31.0486) -> (40.7196, -21.9104) projected
  arc A104 (40.7196, -21.9104) -> (39.937, -20.3236) centre (38.7196, -21.9104) ccw projected
  arc A105 (39.7673, -20.1811) -> (39.937, -20.3236) centre (41.4696, -18.3262) ccw projected
  arc A106 (39.1196, -18.7076) -> (39.7673, -20.1811) centre (41.1196, -18.7076) ccw projected
  line L97 (39.1196, -18.7076) -> (39.1196, -13.7515) projected
  arc A107 (39.7673, -12.2779) -> (39.1196, -13.7515) centre (41.1196, -13.7515) ccw projected
  arc A108 (39.937, -12.1354) -> (39.7673, -12.2779) centre (41.4696, -14.1328) ccw projected
  arc A109 (39.937, -12.1354) -> (40.7196, -10.5486) centre (38.7196, -10.5486) ccw projected
  line L98 (40.7196, -10.5486) -> (40.7196, -1.4104) projected
  arc A110 (40.7196, -1.4104) -> (39.937, 0.1764) centre (38.7196, -1.4104) ccw projected
  arc A111 (39.7673, 0.3189) -> (39.937, 0.1764) centre (41.4696, 2.1738) ccw projected
  arc A112 (39.1196, 1.7924) -> (39.7673, 0.3189) centre (41.1196, 1.7924) ccw projected
  line L99 (39.1196, 1.7924) -> (39.1196, 6.7485) projected
  arc A113 (39.7673, 8.2221) -> (39.1196, 6.7485) centre (41.1196, 6.7485) ccw projected
  arc A114 (39.937, 8.3646) -> (39.7673, 8.2221) centre (41.4696, 6.3672) ccw projected
  arc A115 (39.937, 8.3646) -> (40.7196, 9.9514) centre (38.7196, 9.9514) ccw projected
  line L100 (40.7196, 9.9514) -> (40.7196, 19.0896) projected
  arc A116 (40.7196, 19.0896) -> (39.937, 20.6764) centre (38.7196, 19.0896) ccw projected
  arc A117 (39.7673, 20.8189) -> (39.937, 20.6764) centre (41.4696, 22.6738) ccw projected
  arc A118 (39.1196, 22.2924) -> (39.7673, 20.8189) centre (41.1196, 22.2924) ccw projected
  line L101 (39.1196, 22.2924) -> (39.1196, 27.2485) projected
  arc A119 (39.7673, 28.7221) -> (39.1196, 27.2485) centre (41.1196, 27.2485) ccw projected
  arc A120 (39.937, 28.8646) -> (39.7673, 28.7221) centre (41.4696, 26.8672) ccw projected
  arc A121 (39.937, 28.8646) -> (40.7196, 30.4514) centre (38.7196, 30.4514) ccw projected
  line L102 (40.7196, 30.4514) -> (40.7196, 39.5896) projected
  arc A122 (40.7196, 39.5896) -> (39.937, 41.1764) centre (38.7196, 39.5896) ccw projected
  arc A123 (39.7673, 41.3189) -> (39.937, 41.1764) centre (41.4696, 43.1738) ccw projected
  arc A124 (39.1196, 42.7924) -> (39.7673, 41.3189) centre (41.1196, 42.7924) ccw projected
  line L103 (39.1196, 42.7924) -> (39.1196, 47.7485) projected
  arc A125 (39.7673, 49.2221) -> (39.1196, 47.7485) centre (41.1196, 47.7485) ccw projected
  arc A126 (43.3362, 49.0566) -> (39.7673, 49.2221) centre (41.4696, 47.3672) ccw projected
  arc A127 (43.3362, 49.0566) -> (44.819, 48.3987) centre (44.819, 50.3987) ccw projected
  line L104 (44.819, 48.3987) -> (75, 48.3987) projected
  line L105 (75, 48.3987) -> (75, 184.5) projected
  line L106 (75, 184.5) -> (57.5, 184.5) projected
  line L107 (57.5, 184.5) -> (57.5, 215) projected
  line L108 (57.5, 215) -> (55, 215) projected
  line L109 (55, 215) -> (55, 220) projected
  line L110 (55, 220) -> (24.5, 220) projected
  line L111 (24.5, 220) -> (24.5, 232.5) projected
  line L112 (24.5, 232.5) -> (-24.5, 232.5) projected
  line L113 (-24.5, 232.5) -> (-24.5, 220) projected
  line L114 (-24.5, 220) -> (-55, 220) projected
  line L115 (-55, 220) -> (-55, 215) projected
  line L116 (-55, 215) -> (-78, 215) projected
  line L117 (-78, 215) -> (-78, 46.0635) projected
  line L118 (-78, 46.0635) -> (-75, 46.0635) projected
  line L119 (-55, 215) -> (55, 215)
  line L120 (-24.5, 220) -> (-55, 220) projected
  line L121 (-24.5, 220) -> (-24.5, 215)
  line L122 (24.5, 220) -> (24.5, 215)
  point P0 (0, 0)
  constraints: 6 end point, 2 point on line, 1 horizontal, 1 perpendicular, 1 vertical
extrude "Extrusion3" cut sketch "Sketch3" against normal blind 10 contours L115 L114 L121 L119 | L121 L113 L112 L111 L122 L119 | L122 L110 L109 L119